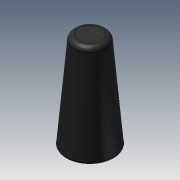
# Autodesk Inventor part: Locking Pin Lever Rubber
Saved by Autodesk Inventor 2011 (Build 150239000, 239)
## iProperties
Created: 2012-11-06
Part Number: Locking Pin Lever Rubber
Material: Rubber
Document SubType Name: Modeling
Designer: Lance
Mass: 0.105163 g
Surface Area: 1.98455 cm^2
Volume: 0.113079 cm^3
Density: 0.93 g/cm^3
Author: Lance
Autodesk Inventor part; units mm, degrees
ref_plane "YZ Plane" through (0, 0, 0) normal (1, 0, 0) x (0, 1, 0)
ref_plane "XZ Plane" through (0, 0, 0) normal (0, 1, 0) x (-1, 0, 0)
ref_plane "XY Plane" through (0, 0, 0) normal (0, 0, 1) x (1, 0, 0)
sketch "Sketch1" plane through (0, 0, 0) normal (0, 1, 0) x (-1, 0, 0)
  line L0 (0, 2) -> (0, 5)
  line L1 (0, 5) -> (-1.6251, 5)
  line L2 (-1.6251, 5) -> (-2.5, -5)
  line L3 (-2.5, -5) -> (-1, -5)
  line L4 (-1, -5) -> (-1, 2)
  line L5 (-1, 2) -> (0, 2)
  point P0 (0, 0)
  point P1 (-2.0626, 0)
  dimension "d0" = 10
  dimension "d1" = 2
  dimension "d2" = 7
  dimension "d3" = 5
  dimension "d4" = 5
  constraints: 12 end point, 3 parallel, 1 horizontal alignment, 1 midpoint, 1 perpendicular, 1 point on line, 1 vertical
  measures "d0" distance between parallel lines of L3 L1
  measures "d1" diameter of L4 L0
  measures "d2" distance between parallel lines of L3 L5
  measures "d3" angle of L4 L2
  measures "d4" diameter of L2.end L0
revolve "Revolution1" add sketch "Sketch1" angle 360 about axis through (0, 0, 2) along (0, 0, 1)
fillet "Fillet1" radius 0.5 1 edges at (-1.6251, 0, 5)
fillet "Fillet2" radius 0.2 1 edges at (-2.5, 0, -5)
body "Solid1"
